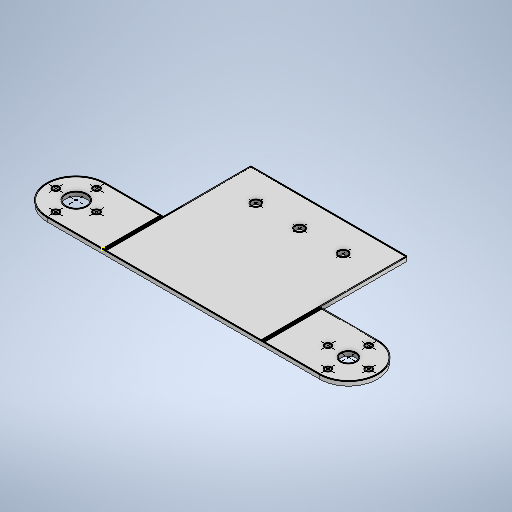
# Autodesk Inventor part: axis_17_bottom_frame
Saved by Autodesk Inventor 2026.1 (Build 301233000, 233)
## iProperties
Created: 2025-08-15
Part Number: axis_17_bottom_frame
Material: Generic
Document SubType Name: Modeling
Designer: LG
Density: 1 g/cm^3
Appearance: Default
Author: LG
Autodesk Inventor part; units mm, degrees
ref_plane "YZ Plane" through (0, 0, 0) normal (1, 0, 0) x (0, 1, 0)
ref_plane "XZ Plane" through (0, 0, 0) normal (0, 1, 0) x (-1, 0, 0)
ref_plane "XY Plane" through (0, 0, 0) normal (0, 0, 1) x (1, 0, 0)
sketch "Sketch1" plane through (0, 0, 0) normal (0, 1, 0) x (-1, 0, 0)
  line L0 (-0.4496, -19.92) -> (-0.4496, 0)
  line L1 (-54.9089, 0) -> (-54.9089, -19.92)
  circle A0 centre (-74.4786, -9.96) radius 2.6
  circle A1 centre (-81.4786, -9.96) radius 1.05
  circle A2 centre (-74.4786, -16.96) radius 1.05
  circle A3 centre (-67.4786, -9.96) radius 1.05
  circle A4 centre (-74.4786, -2.96) radius 1.05
  circle A5 centre (19.12, -9.96) radius 3.6
  circle A6 centre (26.12, -9.96) radius 1.05
  circle A7 centre (19.12, -16.96) radius 1.05
  circle A8 centre (12.12, -9.96) radius 1.05
  circle A9 centre (19.12, -2.96) radius 1.05
  circle A10 centre (-42.6793, -39.96) radius 1.55
  circle A11 centre (-27.6793, -39.96) radius 1.55
  circle A12 centre (-12.6793, -39.96) radius 1.55
  arc A13 (19.19, -19.92) -> (19.19, 0) centre (19.19, -9.96) ccw
  line L2 (19.19, -19.92) -> (-0.8993, -19.92)
  arc A14 (-74.5486, 0) -> (-74.5486, -19.92) centre (-74.5486, -9.96) ccw
  line L3 (-54.4593, -19.92) -> (-74.5486, -19.92)
  line L4 (-54.4593, -50) -> (-54.4593, -19.92)
  line L5 (-0.8993, -19.92) -> (-0.8993, -50)
  line L6 (-0.8993, -50) -> (-54.4593, -50)
  line L7 (-74.5486, 0) -> (19.19, 0)
  line L8 (-55.3586, -19.92) -> (-55.3586, 0)
  line L9 (-54.4593, 0) -> (-54.4593, -19.92)
  line L10 (-0.8993, -19.92) -> (-0.8993, 0)
  line L11 (0, 0) -> (0, -19.92)
  constraints: 24 end point, 15 centre point, 10 equal radius, 10 point on line, 8 vertical, 6 parallel, 4 horizontal, 4 point on circle, 4 tangent, 3 perpendicular, 1 collinear, 49 other
extrude "Extrusion1" add sketch "Sketch1" against normal blind 1.5
body "Solid1"
